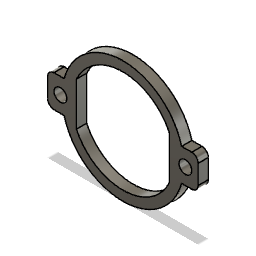
espaciador_rueda_loca_v3 (Autodesk Fusion 360 design; units mm, degrees)
Autodesk Fusion 360 part; units mm, degrees
sketch "Sketch1" plane through (0, 0, 0) normal (0, 0, 1) x (1, 0, 0)
  circle A0 centre (0, 0) radius 16
  line L0 (0, 0) -> (19.5, 0) construction
  circle A1 centre (19.5, 0) radius 2
  line L1 (0, 0) -> (0, 16) construction
  circle A2 centre (-19.5, 0) radius 2
  line L2 (23.5, 5) -> (-23.5, 5)
  line L3 (-23.5, 5) -> (-23.5, -5)
  line L4 (-23.5, -5) -> (23.5, -5)
  line L5 (23.5, -5) -> (23.5, 5)
  line L6 (23.5, 5) -> (-23.5, -5) construction
  line L7 (-23.5, 5) -> (23.5, -5) construction
  circle A3 centre (0, 0) radius 19
  line L8 (-14.5, 5) -> (-24.5, 5)
  line L9 (-24.5, 5) -> (-24.5, -5)
  line L10 (-24.5, -5) -> (-14.5, -5)
  line L11 (-14.5, -5) -> (-14.5, 5)
  line L12 (-14.5, 5) -> (-24.5, -5) construction
  line L13 (-24.5, 5) -> (-14.5, -5) construction
  line L14 (24.5, 5) -> (24.5, -5)
  line L15 (24.5, -5) -> (14.5, -5)
  line L16 (14.5, -5) -> (14.5, 5)
  line L17 (14.5, 5) -> (24.5, 5)
  line L18 (-14.5, -5) -> (-14.5, -6.7639)
  line L19 (-14.5, 5) -> (-14.5, 6.7639)
  line L20 (14.5, 5) -> (14.5, 6.7639)
  line L21 (14.5, -5) -> (14.5, -6.7639)
  point P0 (-19.5, 0)
  dimension "d1" = 32
  dimension "d2" = 19.5
  dimension "d3" = 4
  dimension "d4" = 3
  dimension "d5" = 4
  dimension "d6" = 10
  dimension "d11" = 5
  constraint coincident A0.centre L0.start
  constraint horizontal L0
  constraint coincident L0.end A1.centre
  constraint coincident A0 L1.end
  constraint vertical L1
  constraint symmetric A1 L1 A2
  constraint horizontal L2
  constraint perpendicular L2 L3
  constraint parallel L2 L4
  constraint parallel L3 L5
  constraint coincident L6 A0.centre
  constraint coincident L7 A0.centre
  constraint horizontal L8
  constraint perpendicular L8 L9
  constraint parallel L8 L10
  constraint parallel L9 L11
  constraint coincident L12 P0
  constraint coincident L13 P0
  constraint coincident L2 L8.start
  constraint coincident P0 A2.centre
  constraint symmetric L1 L8.start L16.end
  constraint symmetric L1 L8.end L14.start
  constraint symmetric L1 L9.end L14.end
  constraint symmetric L1 L10.end L15.end
  constraint coincident A0 L18.end
  constraint perpendicular L4 L18
  constraint coincident A0 L19.end
  constraint perpendicular L2 L19
  constraint symmetric L1 L18.end L21.end
  constraint symmetric L1 L19.end L20.end
  measures "d1" diameter of A0
  measures "d2" distance of A0.centre L0.end
  measures "d3" diameter of A1
  measures "d5" distance of L0.end L5
  measures "d6" distance of L2.start L4.end
  measures "d11" distance of P0 L11
extrude "Extrude1" add sketch "Sketch1" along normal blind 3.2 contours A0 L2 A3 L8 L17 | A0 L2 L17 L20 | A0 L2 L8 L19 | A0 A1 L2 L4 A3 L15 L17 | A0 L2 L4 L15 L16 L17 | A0 L2 L4 L8 L10 L11 | A0 A2 L2 L4 A3 L8 L10 | A1 L2 L4 L5 A3 L15 L17 | A0 L4 L15 L21 | A0 L4 L10 L18 | A0 L4 A3 L10 L15 | A2 L2 L3 L4 A3 L8 L10
fillet "Fillet1" radius 2 4 edges at (-23.5, -5, 1.6) (-23.5, 5, 1.6) (23.5, -5, 1.6) (23.5, 5, 1.6)
equation "d2 = ( 39 / 2 ) * 1 mm"
